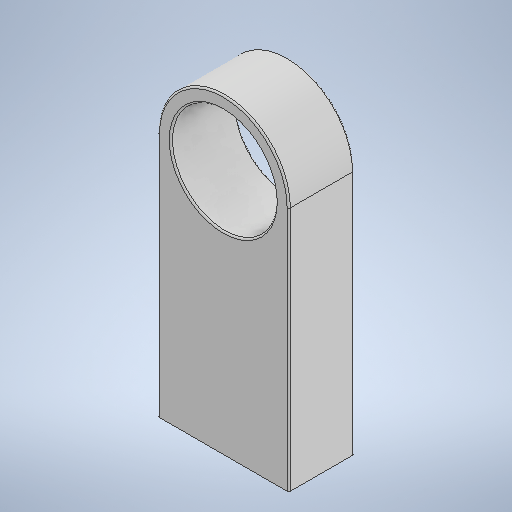
# Autodesk Inventor part: Steering Support
Saved by Autodesk Inventor 2025.2 (Build 292293000, 293)
## iProperties
Created: 2025-02-04
Part Number: Steering Support
Material: Generic
Document SubType Name: Modeling
Designer: eason
Density: 1 g/cm^3
Appearance: Default
Author: eason
Autodesk Inventor part; units mm, degrees
ref_plane "YZ Plane" through (0, 0, 0) normal (1, 0, 0) x (0, 1, 0)
ref_plane "XZ Plane" through (0, 0, 0) normal (0, 1, 0) x (-1, 0, 0)
ref_plane "XY Plane" through (0, 0, 0) normal (0, 0, 1) x (1, 0, 0)
sketch "Sketch1" plane through (0, 0, 0) normal (0, 0, 1) x (1, 0, 0)
  circle A0 centre (0, 0) radius 16
  arc A1 (20, 0) -> (-20, 0) centre (0, 0) ccw
  line L0 (20, 0) -> (20, -75)
  line L1 (20, -75) -> (-20, -75)
  line L2 (-20, -75) -> (-20, 0)
  line L3 (-28, 0) -> (28, 0) projected
  dimension "d0" = 32
  dimension "d1" = 40
  dimension "d2" = 75
  constraints: 6 end point, 2 centre point, 2 coincident, 2 point on circle, 2 point on line, 2 tangent, 1 parallel
  measures "d0" diameter of A0
  measures "d1" diameter of A1
  measures "d2" distance between parallel lines of L3 L1
extrude "Extrusion1" add sketch "Sketch1" along normal blind 20 contours L3 L0 L1 L2 A0 | A0 L3 A1
sketch "Sketch2" plane through (-20, -75, 0) normal (0, -1, 0) x (1, 0, 0)
  circle A0 centre (30, 10) radius 5
  circle A1 centre (10, 10) radius 5
  line L0 (40, 0) -> (40, 20) projected
  line L1 (40, 10) -> (0, 10) construction
  line L2 (0, 0) -> (0, 20) projected
  point P0 (20, 0)
  dimension "d5" = 10
  dimension "d6" = 10
  dimension "d7" = 20
  dimension "d8" = 40
  dimension "d9" = 10
  constraints: 2 centre point, 2 end point, 2 midpoint, 2 point on line
  measures "d5" diameter of A0
  measures "d6" diameter of A1
  measures "d7" distance of A1.centre A0.centre
  measures "d8" distance between parallel lines of L2 L0
  measures "d9" distance from line of L0 A0.centre
extrude "Extrusion2" cut sketch "Sketch2" against normal blind 40
fillet "Fillet1" radius 0.5 10 edges at (5, -75, 10) (-15, -75, 10) (-16, 0, 20) (-16, 0, 0) (-20, -37.5, 20) (20, -37.5, 20) (0, 20, 20) (-20, -37.5, 0) (20, -37.5, 0) (0, 20, 0)
thread "Thread1" size "M10x1.5" class "6H" standard "ANSI Metric M Profile" full length
thread "Thread2" size "M10x1.5" class "6H" standard "ANSI Metric M Profile" full length
body "Solid1"
